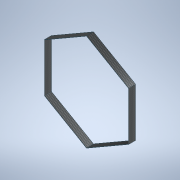
# Autodesk Inventor part: Wallmesh
Saved by Autodesk Inventor 2020.3 (Build 243373000, 373)
## iProperties
Created: 2020-07-07
Part Number: Wallmesh
Material: Generic
Document SubType Name: Modeling
Designer: Bruno
Density: 1 g/cm^3
Appearance: Expanded Metal 04
Author: Bruno
Autodesk Inventor part; units mm, degrees
ref_plane "YZ Plane" through (0, 0, 0) normal (1, 0, 0) x (0, 1, 0)
ref_plane "XZ Plane" through (0, 0, 0) normal (0, 1, 0) x (-1, 0, 0)
ref_plane "Work Plane1" through (0, 0, 0) normal (0, 0, 1) x (1, 0, 0)
sketch "Sketch1" plane through (0, 0, 0) normal (0, 0, 1) x (1, 0, 0)
  line L0 (300, -173.2051) -> (0, -346.4102)
  line L1 (0, -346.4102) -> (-300, -173.2051)
  line L2 (-300, -173.2051) -> (-300, 173.2051)
  line L3 (-300, 173.2051) -> (0, 346.4102)
  line L4 (0, 346.4102) -> (300, 173.2051)
  line L5 (300, 173.2051) -> (300, -173.2051)
  line L6 (302, 174.3598) -> (302, -174.3598)
  line L7 (302, -174.3598) -> (0, -348.7196)
  line L8 (0, -348.7196) -> (-302, -174.3598)
  line L9 (-302, -174.3598) -> (-302, 174.3598)
  line L10 (-302, 174.3598) -> (0, 348.7196)
  line L11 (0, 348.7196) -> (302, 174.3598)
  point P0 (0, 0)
  point P1 (0, 0)
  point P2 (0, 0)
  dimension "d0" = 302
  dimension "d1" = 300
  constraints: 24 end point, 2 coincident, 2 vertical, 26 other
  measures "d0" distance from line of point (0, 0) L6
  measures "d1" distance from line of point (0, 0) L5
extrude "Extrusion1" add sketch "Sketch1" along normal blind 50
body "Solid1"
